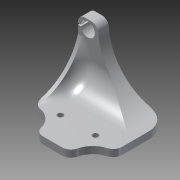
# Autodesk Inventor part: top-left bracket - 2hole
Saved by Autodesk Inventor 2015 SP1 (Build 190203100, 203)
## iProperties
Created: 2015-01-03
Part Number: top-left bracket - 2hole
Material: ABS Plastic
Document SubType Name: Modeling
Designer: Luna
Density: 1.06 g/cm^3
Appearance: Smooth - White
Mass: 2.06395 g
Surface Area: 14.6209 cm^2
Volume: 1.94712 cm^3
Author: Luna
Autodesk Inventor part; units mm, degrees
ref_plane "YZ Plane" through (0, 0, 0) normal (1, 0, 0) x (0, 1, 0)
ref_plane "XZ Plane" through (0, 0, 0) normal (0, 1, 0) x (-1, 0, 0)
ref_plane "XY Plane" through (0, 0, 0) normal (0, 0, 1) x (1, 0, 0)
sketch "Sketch3" plane through (0, 0, 0) normal (0, 0, 1) x (1, 0, 0)
  line L0 (-7, 0) -> (7, 0) construction
  line L1 (-7, 0) -> (7, 0) construction
  line L2 (-9, -2) -> (9, -2)
  line L3 (9, -2) -> (9, 2)
  line L4 (9, 2) -> (-9, 2)
  line L5 (-9, 2) -> (-9, -2)
  line L6 (-9, -2) -> (9, 2) construction
  line L7 (9, -2) -> (-9, 2) construction
  line L8 (0, 0) -> (0, -13) construction
  line L9 (-2, 2) -> (2, 2)
  line L10 (2, 2) -> (2, -15)
  line L11 (2, -15) -> (-2, -15)
  line L12 (-2, -15) -> (-2, 2)
  line L13 (17, -10) -> (-17, -10)
  line L14 (-17, -10) -> (-17, 10)
  line L15 (-17, 10) -> (17, 10)
  line L16 (17, 10) -> (17, -10)
  line L17 (10, -23) -> (10, 10)
  line L18 (10, 10) -> (-10, 10)
  line L19 (-10, 10) -> (-10, -23)
  line L20 (-10, -23) -> (10, -23)
  point P0 (0, -6.5)
  point P1 (0, 2)
  point P2 (0, -6.5)
  point P3 (0, 2)
  dimension "d31" = 18
  dimension "d32" = 4
  dimension "d33" = 4
  dimension "d34" = 17
  dimension "d35" = 8
  dimension "d36" = 8
  constraints: 40 end point, 8 parallel, 6 midpoint, 4 perpendicular, 2 horizontal, 1 coincident, 1 vertical alignment, 6 other
  measures "d31" distance of L4.end L3.end
  measures "d32" distance of L3.end L2.end
  measures "d33" distance of L10.end L11.end
  measures "d34" distance of L9.end L10.end
  measures "d35" distance between parallel lines of L2 L13
  measures "d36" distance between parallel lines of L10 L17
extrude "back plate Extrusion2" add sketch "Sketch3" against normal blind 4
sketch "Sketch4" plane through (-17, 10, 0) normal (0, 1, 0) x (1, 0, 0)
  line L0 (34, 0) -> (0, 0) projected
  line L1 (34, 0) -> (34, 4) projected
  line L2 (0, 4) -> (34, 4) projected
  line L3 (0, 0) -> (0, 4) projected
  point P0 (17, 0)
extrude "Extrusion3" add sketch "Sketch4" along normal blind 11.5
sketch "Sketch9" plane through (-17, 21.5, 0) normal (0, 1, 0) x (1, 0, 0)
  line L0 (39, -41.948) -> (39, -44) projected
  line L1 (34, 4) -> (39, 4)
  line L2 (39, 4) -> (39, 0)
  line L3 (39, 0) -> (34, 0)
  line L4 (34, 0) -> (34, 4)
  point P0 (17, 0)
  dimension "d58" = 4
  constraints: 8 end point, 2 parallel, 1 horizontal, 1 perpendicular, 1 point on line
  measures "d58" distance between parallel lines of L1 L3
extrude "Extrusion6" add sketch "Sketch9" against normal blind 6
sketch "Sketch10" plane through (-17, 21.5, 0) normal (0, 1, 0) x (1, 0, 0)
  line L0 (39, -41.948) -> (39, -44) projected
  line L1 (-3.3, -41.948) -> (-3.3, -44) projected
  arc A0 (-3.3, -44) -> (0.7, -48) centre (0.7, -44) ccw projected
  line L2 (2.35, -48) -> (0.7, -48) projected
  arc A1 (2.35, -48) -> (6.35, -44) centre (2.35, -44) ccw projected
  line L3 (6.35, -44) -> (6.35, -27.15) projected
  arc A2 (29.35, -27.15) -> (6.35, -27.15) centre (17.85, -27.15) ccw projected
  line L4 (29.35, -27.15) -> (29.35, -44) projected
  arc A3 (29.35, -44) -> (33.35, -48) centre (33.35, -44) ccw projected
  line L5 (35, -48) -> (33.35, -48) projected
  arc A4 (35, -48) -> (39, -44) centre (35, -44) ccw projected
  line L6 (41, -27.65) -> (41, -28.6815) projected
  line L7 (41, -27.65) -> (39.3186, -27.65) projected
  arc A5 (39.3186, -26.65) -> (39.3186, -27.65) centre (35.35, -27.15) ccw projected
  line L8 (39.3186, -26.65) -> (41, -26.65) projected
  circle A6 centre (2.35, -42.65) radius 1.6 projected
  circle A7 centre (33.35, -11.65) radius 1.6 projected
  circle A8 centre (2.35, -11.65) radius 1.6 projected
  circle A9 centre (33.35, -42.65) radius 1.6 projected
  line L9 (34, 0) -> (27, 0) projected
  line L10 (29.35, 0) -> (39, 0)
  line L11 (39, 0) -> (39, -48)
  line L12 (39, -48) -> (29.35, -48)
  line L13 (29.35, -48) -> (29.35, 0)
  line L14 (39, -32.15) -> (41, -32.15)
  line L15 (41, -32.15) -> (41, -22.15)
  line L16 (41, -22.15) -> (39, -22.15)
  line L17 (39, -22.15) -> (39, -32.15)
  line L18 (41, 4) -> (41, -26.65) projected
  line L19 (-5.3, 4) -> (41, 4) projected
  arc A10 (40.1111, -34.5777) -> (41, -28.6815) centre (21, -28.6815) ccw projected
  line L20 (-5.3, 4) -> (-5.3, -28.6815) projected
  arc A11 (-5.3, -28.6815) -> (-4.4111, -34.5777) centre (14.7, -28.6815) ccw projected
  arc A12 (-3.3, -41.948) -> (-4.4111, -34.5777) centre (-28.3, -41.948) ccw projected
  arc A13 (40.1111, -34.5777) -> (39, -41.948) centre (64, -41.948) ccw projected
  point P0 (17, 0)
  dimension "d63" = 5.5
  dimension "d64" = 20.35
  constraints: 16 end point, 4 parallel, 2 horizontal, 2 perpendicular, 1 point on line
  measures "d63" distance between parallel lines of L7 L16
  measures "d64" distance between parallel lines of L7 L12
extrude "Extrusion7" add sketch "Sketch10" against normal blind 6 contours L0 A4 L5 A3 L4 L13 L9 L10 L11 A5 | L11 L12 A4 | L11 A5 L7 L6 A10 L14 | L11 A5 L8 L15 L7 | A5 L11 | A10 L15 L14 | L12 L13 A3 | L11 L16 L15 L8 A5 | A7 | A9
sketch "Sketch11" plane through (-17, 21.5, 0) normal (0, 1, 0) x (1, 0, 0)
  circle A0 centre (35.35, -27.15) radius 4 projected
  point P0 (17, 0)
hole "Hole4" at (18.35, 21.5, 27.15) direction (0, -1, 0) diameter 8 end through all
sketch "Sketch12" plane through (24, 21.5, 32.15) normal (1, 0, 0) x (0, 0, -1)
  line L0 (4.5, 0) -> (5.5, 0)
  line L1 (5.5, 0) -> (5.5, -6)
  line L2 (5.5, -6) -> (4.5, -6)
  line L3 (4.5, -6) -> (4.5, 0)
  line L4 (0, 0) -> (10, 0) projected
  point P0 (32.15, -21.5)
  point P1 (5, 0)
  point P2 (5, 0)
  point P3 (5, 0)
  dimension "d74" = 1
  dimension "d75" = 6
  constraints: 8 end point, 3 midpoint, 2 coincident, 2 parallel, 1 horizontal, 1 perpendicular
  measures "d74" distance of L1.end L2.end
  measures "d75" distance of L0.end L1.end
extrude "Extrusion8" cut sketch "Sketch12" against normal blind 6
sketch "Sketch13" plane through (12.35, 21.5, 48) normal (0, 0, 1) x (1, 0, 0)
  line L0 (9.65, 0) -> (0, 0) projected
  line L1 (0, 0) -> (0, -6) projected
  line L2 (9.65, -6) -> (0, -6) projected
  line L3 (9.65, 0) -> (9.65, -6) projected
  point P0 (-12.35, -21.5)
extrude "Extrusion9" cut sketch "Sketch13" against normal blind 15.85
fillet "Fillet4" radius 4 2 edges at (12.35, 18.5, 32.15) (24, 18.5, 32.15)
sketch "Sketch14" plane through (17, 15.5, 0) normal (1, 0, 0) x (0, 0, -1)
  line L0 (4, -25.5) -> (4, 0) projected
  line L1 (4, 0) -> (0, 0) projected
  line L2 (0, -25.5) -> (0, 0) projected
  line L3 (0, -25.5) -> (4, -25.5) projected
  point P0 (0, -15.5)
extrude "Extrusion10" add sketch "Sketch14" along normal blind 5
sketch "Sketch16" plane through (-17, 21.5, -4) normal (-1, 0, 0) x (0, 0, 1)
  line L0 (4, -31.5) -> (4, 0) projected
  line L1 (0, 0) -> (4, 0) projected
  line L2 (0, -31.5) -> (0, 0) projected
  line L3 (4, -31.5) -> (0, -31.5) projected
  point P0 (4, -21.5)
extrude "Extrusion12" add sketch "Sketch16" along normal blind 5.25
sketch "Sketch17" plane through (22, -10, -4) normal (1, 0, 0) x (0, 0, -1)
  line L0 (0, 31.5) -> (-26.15, 31.5) projected
  line L1 (-26.15, 31.5) -> (-26.15, 25.5) projected
  line L2 (-4, 25.5) -> (-26.15, 25.5) projected
  line L3 (-4, 25.5) -> (-4, 0) projected
  line L4 (-4, 0) -> (0, 0) projected
  line L5 (0, 31.5) -> (0, 0) projected
  arc A0 (-4, 0) -> (-26.15, 25.5) centre (-33.794, -3.5098) ccw
  point P0 (-4, 10)
  dimension "d96" = 30
  constraints: 2 point on circle, 1 centre point
  measures "d96" radius of A0
extrude "Extrusion13" add sketch "Sketch17" along normal blind 2
fillet "Fillet13" radius 30 1 edges at (12.35, 18.5, 0)
fillet "Fillet14" radius 13 1 edges at (2.2002, 15.5, 0)
fillet "Fillet15" radius 12 3 edges at (-10, -10, -2) (10, -10, -2) (-22.25, 21.5, -2)
fillet "Fillet16" radius 5 4 edges at (-22.25, -10, -2) (-10, -23, -2) (10, -23, -2) (24, -10, -2)
fillet "Fillet17" radius 7 3 edges at (22, -3.3834, 0) (22, 15.5, 17.575) (22, 11.6924, 3.8076)
sketch "Sketch19" plane through (0, 0, 0) normal (0, 0, 1) x (1, 0, 0)
  circle A0 centre (-9, -7.5) radius 2 projected
  circle A1 centre (11, -7.5) radius 2 projected
  point P0 (0, 0)
hole "Hole5" at (-9, -7.5, 0) at (11, -7.5, 0) direction (0, 0, -1) diameter 3.2 end through all
mirror "Mirror1" about plane through (0, 0, 0) normal (1, 0, 0) remove original yes
body "Solid2"
